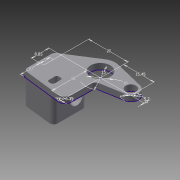
# Autodesk Inventor part: bowden_tube_holder
Saved by Autodesk Inventor 2015 (Build 190159000, 159)
## iProperties
Created: 2015-01-19
Part Number: bowden_tube_holder
Material: Generic
Document SubType Name: Modeling
Designer: Justin
Density: 1 g/cm^3
Appearance: Default
Author: Justin
Autodesk Inventor part; units mm, degrees
ref_plane "YZ Plane" through (0, 0, 0) normal (1, 0, 0) x (0, 1, 0)
ref_plane "XZ Plane" through (0, 0, 0) normal (0, 1, 0) x (-1, 0, 0)
ref_plane "XY Plane" through (0, 0, 0) normal (0, 0, 1) x (1, 0, 0)
sketch "Sketch1" plane through (0, 0, 0) normal (0, 0, 1) x (1, 0, 0)
  circle A0 centre (0, 0) radius 5
  circle A1 centre (15.45, 0) radius 2.6
  arc A2 (16.1104, -3.7929) -> (16.3595, 3.741) centre (15.45, 0) ccw
  arc A3 (1.7718, 7.2877) -> (-3.175, -6.7948) centre (0, 0) ccw
  line L0 (1.7718, 7.2877) -> (16.3595, 3.741)
  arc A4 (-3.175, -18) -> (3.175, -18) centre (0, -18) ccw
  line L1 (3.175, -18) -> (3.175, -6.045)
  line L2 (-3.175, -6.7948) -> (-3.175, -18)
  line L3 (-20, -8.85) -> (-20, -3.85)
  line L4 (-20, -8.85) -> (-20, -18.85)
  line L5 (-20, -3.85) -> (-4.0301, 6.3252)
  line L6 (-20, -3.85) -> (-6.4364, -3.85)
  line L7 (-20, -18.85) -> (-0.37, -21.1534)
  line L8 (16.1104, -3.7929) -> (3.175, -6.045)
  line L9 (-3.175, -18) -> (-3.175, -20.8242)
  point P0 (-20, -5.6718)
  dimension "d0" = 15.45
  dimension "d1" = 5.2
  dimension "d2" = 10
  dimension "d3" = 0
  dimension "d4" = 7.7
  dimension "d5" = 15
  dimension "d6" = 6.35
  dimension "d7" = 0
  dimension "d9" = 18
  dimension "d21" = 8.85
  dimension "d22" = 20
  dimension "d23" = 5
  dimension "d24" = 10
  constraints: 20 end point, 10 point on circle, 6 tangent, 5 centre point, 5 vertical, 3 coincident, 2 point on line, 1 horizontal, 1 other
  measures "d0" distance of A1.centre point (0, 0)
  measures "d1" diameter of A1
  measures "d2" diameter of A0
  measures "d3" vertical distance of point (0, 0) A1.centre
  measures "d4" diameter of A2
  measures "d5" diameter of A3
  measures "d6" diameter of A4
  measures "d7" horizontal distance of A4.centre point (0, 0)
  measures "d9" distance of A4.centre point (0, 0)
  measures "d21" vertical distance of point (0, 0) L3.start
  measures "d22" horizontal distance of A0.centre L3.start
  measures "d23" distance of L3.start L3.end
  measures "d24" distance of L3.start L4.end
extrude "Extrusion3" add sketch "Sketch1" along normal blind 3
fillet "Fillet7" radius 2 1 edges at (3.175, -6.045, 1.5)
extrude "Extrusion6" add sketch "Sketch1" against normal blind 12.3 contours A3 L2 L9 L7 L4 L3 L6
sketch "Sketch5" plane through (-20, -18.85, 3) normal (-1, 0, 0) x (0, 0, 1)
  line L0 (-3, 26.35) -> (0, 26.35) projected
  line L1 (0, 15) -> (0, 0) projected
  circle A0 centre (-9.15, 10) radius 3.15
  line L2 (-3, -1.9742) -> (-3, 12.0552) projected
  point P0 (-3, 18.85)
  point P1 (-3, 13.1782)
  point P2 (-3, 10)
  dimension "d43" = 6.3
  dimension "d44" = 0
  dimension "d45" = 6.15
  constraints: 1 centre point
  measures "d43" diameter of A0
  measures "d44" vertical distance of point (-3, 10) A0.centre
  measures "d45" distance from line of L2 A0.centre
sketch "Sketch6" plane through (0, 0, 3) normal (0, 0, 1) x (1, 0, 0)
  line L0 (-20, -12) -> (-3.175, -12) projected
  circle A0 centre (0, 0) radius 5 projected
  circle A1 centre (15.45, 0) radius 2.6 projected
  line L1 (-4.0301, 6.3252) -> (-20, -3.85) projected
  line L2 (-20, -3.85) -> (-20, -18.85) projected
  line L3 (-20, -18.85) -> (-0.37, -21.1534) projected
  arc A2 (-0.37, -21.1534) -> (3.175, -18) centre (0, -18) ccw projected
  line L4 (3.175, -18) -> (3.175, -7.7269) projected
  arc A3 (4.832, -5.7565) -> (3.175, -7.7269) centre (5.175, -7.7269) ccw projected
  line L5 (4.832, -5.7565) -> (16.1104, -3.7929) projected
  arc A4 (16.1104, -3.7929) -> (16.3595, 3.741) centre (15.45, 0) ccw projected
  line L6 (16.3595, 3.741) -> (1.7718, 7.2877) projected
  arc A5 (1.7718, 7.2877) -> (-4.0301, 6.3252) centre (0, 0) ccw projected
  line L7 (-20, -5.7) -> (-4.8744, -5.7) projected
  line L8 (-3.175, -20.8242) -> (-3.175, -6.7948) projected
  line L9 (-3.175, -6.7948) -> (-3.175, -20.8242) projected
  line L10 (-9.175, -18) -> (-6.175, -18)
  line L11 (-6.175, -18) -> (-6.175, -13)
  line L12 (-6.175, -13) -> (-9.175, -13)
  line L13 (-9.175, -13) -> (-9.175, -18)
  dimension "d55" = 5
  dimension "d56" = 3
  dimension "d57" = 3
  dimension "d58" = 1
  constraints: 8 end point, 2 parallel, 1 horizontal, 1 perpendicular
  measures "d55" distance of L12.end L10.start
  measures "d56" distance of L11.end L12.end
  measures "d57" distance between parallel lines of L8 L11
  measures "d58" distance between parallel lines of L0 L12
extrude "Extrusion8" cut sketch "Sketch6" against normal up to next contours L13 L12 L11 L10
fillet "Fillet8" radius 2 1 edges at (-20, -18.85, -4.65)
fillet "Fillet9" radius 2 1 edges at (-20, -3.85, -6.15)
fillet "Fillet10" radius 1 1 edges at (-6.175, -18, -4.65)
fillet "Fillet11" radius 1 1 edges at (-9.175, -18, -4.65)
fillet "Fillet12" radius 1 1 edges at (-9.175, -13, -4.65)
fillet "Fillet13" radius 1 1 edges at (-6.175, -13, -4.65)
fillet "Fillet14" radius 2 1 edges at (-3.175, -20.8242, -6.15)
fillet "Fillet18" radius 2 1 edges at (-20, -3.85, 1.5)
sketch "Sketch8" plane through (0, 0, -12.3) normal (0, 0, -1) x (-1, 0, 0)
  line L0 (18, -3.85) -> (6.4364, -3.85) projected
  line L1 (6.175, -17) -> (6.175, -14) projected
  arc A0 (7.175, -13) -> (6.175, -14) centre (7.175, -14) ccw projected
  line L2 (7.175, -13) -> (8.175, -13) projected
  arc A1 (9.175, -14) -> (8.175, -13) centre (8.175, -14) ccw projected
  line L3 (9.175, -14) -> (9.175, -17) projected
  arc A2 (8.175, -18) -> (9.175, -17) centre (8.175, -17) ccw projected
  line L4 (8.175, -18) -> (7.175, -18) projected
  arc A3 (6.175, -17) -> (7.175, -18) centre (7.175, -17) ccw projected
  arc A4 (3.175, -18.5758) -> (5.4081, -20.5622) centre (5.175, -18.5758) ccw projected
  line L5 (5.4081, -20.5622) -> (18.2331, -19.0573) projected
  arc A5 (18.2331, -19.0573) -> (20, -17.071) centre (18, -17.071) ccw projected
  line L6 (20, -17.071) -> (20, -5.85) projected
  arc A6 (20, -5.85) -> (18, -3.85) centre (18, -5.85) ccw projected
  line L7 (18, -3.85) -> (6.4364, -3.85) projected
  arc A7 (3.175, -6.7948) -> (6.4364, -3.85) centre (0, 0) ccw projected
  line L8 (3.175, -6.7948) -> (3.175, -18.5758) projected
  line L9 (19.9944, -5.7) -> (4.8744, -5.7) projected
  circle A8 centre (0, 0) radius 7.5
  line L10 (3.175, -6.7948) -> (3.175, -3.85)
  line L11 (3.175, -3.85) -> (6.4364, -3.85)
  constraints: 4 end point, 1 centre point, 1 coincident, 1 concentric, 1 perpendicular, 1 vertical
extrude "Extrusion9" add sketch "Sketch8" against normal up to surface (12.3 mm away) contours A7 L10 L11
extrude "Extrusion10" cut sketch "Sketch5" against normal up to next
fillet "Fillet19" radius 2 1 edges at (-3.175, -3.85, -6.15)
body "Solid2"
